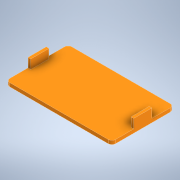
# Autodesk Inventor part: BatteryPlate
Saved by Autodesk Inventor 2021 (Build 250183000, 183)
## iProperties
Created: 2021-05-13
Part Number: BatteryPlate
Material: Generic
Document SubType Name: Modeling
Designer: ermoz
Density: 1 g/cm^3
Appearance: Default
Author: ermoz
Autodesk Inventor part; units mm, degrees
ref_plane "YZ Plane" through (0, 0, 0) normal (1, 0, 0) x (0, 1, 0)
ref_plane "XZ Plane" through (0, 0, 0) normal (0, 1, 0) x (-1, 0, 0)
ref_plane "XY Plane" through (0, 0, 0) normal (0, 0, 1) x (1, 0, 0)
sketch "Sketch1" plane through (0, 0, 0) normal (0, 1, 0) x (-1, 0, 0)
  line L0 (-29, -17) -> (29, -17)
  line L1 (29, -17) -> (29, 17)
  line L2 (29, 17) -> (-29, 17)
  line L3 (-29, 17) -> (-29, -17)
  line L4 (-29, -17) -> (29, 17) construction
  line L5 (29, -17) -> (-29, 17) construction
  point P0 (0, 0)
  dimension "d0" = 34
  dimension "d1" = 58
  constraints: 12 end point, 2 midpoint, 2 parallel, 1 horizontal, 1 perpendicular
  measures "d0" distance of L0.end L1.end
  measures "d1" distance of L1.end L2.end
extrude "Extrusion1" add sketch "Sketch1" along normal blind 2
sketch "Sketch2" plane through (0, 2, 0) normal (0, 1, 0) x (1, 0, 0)
  line L0 (-29, 17) -> (-29, -17) projected
  line L1 (-29, 5) -> (-27.5, 5)
  line L2 (-27.5, 5) -> (-27.5, -5)
  line L3 (-27.5, -5) -> (-29, -5)
  line L4 (-29, -5) -> (-29, 5)
  line L5 (0, 0) -> (0, 9.1837)
  line L6 (0, 0) -> (-7.2938, 0)
  line L7 (29, 5) -> (27.5, 5)
  line L8 (27.5, 5) -> (27.5, -5)
  line L9 (27.5, -5) -> (29, -5)
  line L10 (29, -5) -> (29, 5)
  dimension "d4" = 1.5
  dimension "d5" = 10
  constraints: 20 end point, 4 symmetric about line, 2 horizontal, 2 parallel, 1 perpendicular, 1 point on line, 1 vertical, 1 other
  measures "d4" distance of L1.start L1.end
  measures "d5" distance of L1.end L2.end
extrude "Extrusion2" add sketch "Sketch2" along normal blind 5
fillet "Fillet1" radius 2 4 edges at (29, 1, 17) (29, 1, -17) (-29, 1, -17) (-29, 1, 17)
body "Solid1"
